Autodesk Fusion 360 part; units mm, degrees
(part 2 of 2)
  constraint tangent L245 A257
  constraint tangent A258 L248
  constraint tangent A259 L249
  constraint coincident L250.end L252
  constraint coincident L243 L250.start
  constraint horizontal L251
  constraint tangent L242 A260
  constraint tangent L251 A261
  constraint tangent L243 A261
  constraint tangent L251 A262
  constraint tangent L252 A262
  constraint tangent L247 A263
  constraint tangent L243 A263
  constraint tangent L247 A264
  constraint tangent L252 A264
  constraint coincident L252 L253.end
  constraint coincident L243 L253.start
  measures "d1" diameter of A0
  measures "d2" diameter of A1
  measures "d3" diameter of A2
  measures "d4" diameter of A3
  measures "d5" diameter of A4
  measures "d9" diameter of A111
  measures "d12" diameter of A112
  measures "d367" diameter of A246
  measures "d368" diameter of A247
  measures "d369" diameter of A248
  measures "d370" diameter of A249
extrude "Extrude1" add sketch "mriya-classic-fdm-301645" along normal blind 12.1 contours L176 L177 L198 A202 L199 A203 L200 A204 L201 A205 L202 A206 L203 A207 L204 A208 L205 A209 L206 A210 L207 L208 A212 L209 A213 L210 A214 L211 A215 L212 A216 L213 A217 L214 A218 L215 A219 L216 A220 L217 A221 L218 A222 L219 A223 L220 L221 L222 L223 L224 L225 L226 L227 L228 L229 L230 L231 L232 L233 L234 L235 L236 L237 L238 L239 L240 L241 A224 A225 A227 A228 A229 A230 A231 A232 A233 A234 A235 A236 A237 A238 A239 A240 A241 A242 A243 A244 A245 makes body 1
extrude "Extrude2" add sketch "mriya-classic-fdm-301645" along normal blind 18.6 contours L176 L177 L207 A211 L208 L235 L236 A226 bodies 1
extrude "Extrude3" add sketch "mriya-classic-fdm-301645" along normal blind 5.2 contours A114 | A115 | A116 | A117 | L198 A202 L199 A203 L200 A204 L201 A205 L202 A206 L203 A207 L204 A208 L205 A209 L206 A210 L207 L208 A212 L209 A213 L210 A214 L211 A215 L212 A216 L213 A217 L214 A218 L215 A219 L216 A220 L217 A221 L218 A222 L219 A223 L242 L244 L245 A250 A251 A252 A257 A260 | L207 A211 L208 L244 L245 A250 A251 A257 | L207 L242 A252 A260 bodies 1
extrude "Extrude13" add sketch "mriya-classic-fdm-301645" along normal blind 3.2 contours A2 | L108 L109 A118 A119 A120 L183 L184 A253 | A121 L110 A122 L111 A123 L178 L179 A254 | A124 L112 A125 L113 A126 L114 A127 L115 | A128 L116 A129 L117 A130 L118 A131 L119 | A132 L120 A133 A134 L121 L185 L186 L187 A194 A195 | A135 L122 A136 A137 L123 L180 L181 L182 A196 A197 | A138 L124 A139 L125 A140 L126 A141 L127 | A142 L128 A143 L129 A144 L130 A145 L131 | A146 L132 A147 L133 A148 L134 A149 L135 | A150 L136 A151 L137 A152 L138 A153 L139 | A154 L140 A155 L141 A156 L142 A157 L143 | A158 L144 A159 L145 A160 L146 A161 L147 | A162 L148 A163 L149 A164 L150 A165 L151 | A166 L152 A167 L153 A168 L190 L191 L192 A198 A199 | A169 L154 A170 L155 A171 L156 A172 L157 | A173 L158 A174 L159 A175 L195 L196 L197 A200 A201 | A176 L160 A177 L161 A178 L162 A179 L163 | A180 A181 L164 A182 L165 L193 L194 A256 | A183 L166 A184 L167 A185 L168 A186 L169 | A187 A188 L170 A189 L171 L188 L189 A255 | A190 L172 A191 L173 A192 L174 A193 L175 bodies 1
extrude "Extrude14" add sketch "mriya-classic-fdm-301645" along normal blind 3.2 contours A0 | A1 | A3 | A4 bodies 1
extrude "Extrude6" add sketch "mriya-classic-fdm-301645" along normal blind 1 from surface at 15.8 contours L207 A211 L208 L244 L245 A250 A251 A257 bodies 1
extrude "Extrude12" add sketch "mriya-classic-fdm-301645" along normal blind 1 from surface at 9.2 contours L207 L242 A252 A260 bodies 1
extrude "Extrude21" add sketch "mriya-classic-fdm-301645" along normal blind 2.7 contours L243 L251 L252 A261 A262 L253 | L243 L247 L250 L252 A263 A264 bodies 1
extrude "Extrude19" add sketch "mriya-classic-fdm-301645" along normal blind 1.4 contours L243 L250 L252 L253 bodies 1
sketch "power switch" plane through (-4.4, 0, 0) normal (1, 0, 0) x (0, 1, 0)
  line L0 (1.7932, 0) -> (76.6932, 0)
  line L1 (76.6932, 0) -> (76.6932, 18.6)
  line L2 (76.6932, 18.6) -> (19.2932, 18.6)
  line L3 (19.2932, 18.6) -> (19.2932, 12.1)
  line L4 (19.2932, 12.1) -> (1.7932, 12.1)
  line L5 (1.7932, 12.1) -> (1.7932, 0)
  line L6 (23.9932, 5.95) -> (23.9932, 10.8)
  line L7 (37.3932, 5.55) -> (24.3932, 5.55)
  arc A0 (37.7932, 10.8) -> (37.3932, 11.2) centre (37.3932, 10.8) ccw
  line L8 (36.0932, 9.85) -> (36.0932, 6.9)
  line L9 (25.6932, 9.85) -> (36.0932, 9.85)
  line L10 (36.0932, 6.9) -> (25.6932, 6.9)
  line L11 (25.6932, 6.9) -> (25.6932, 9.85)
  line L12 (24.3932, 11.2) -> (37.3932, 11.2)
  arc A1 (23.9932, 5.95) -> (24.3932, 5.55) centre (24.3932, 5.95) ccw
  arc A2 (37.3932, 5.55) -> (37.7932, 5.95) centre (37.3932, 5.95) ccw
  line L13 (37.7932, 10.8) -> (37.7932, 5.95)
  arc A3 (24.3932, 11.2) -> (23.9932, 10.8) centre (24.3932, 10.8) ccw
  constraint perpendicular L10 L11
  constraint vertical L11
  constraint perpendicular L9 L11
  constraint vertical L8
  constraint tangent A0 L12
  constraint tangent A0 L13
  constraint tangent A2 L13
  constraint tangent L7 A2
  constraint tangent L7 A1
  constraint tangent L6 A1
  constraint tangent L6 A3
  constraint tangent L12 A3
extrude "Extrude8" cut sketch "power switch" against normal blind 2.5 contours L8 L9 L10 L11 bodies 1
extrude "Extrude9" cut sketch "power switch" against normal blind 1 contours L6 L7 A0 L12 A1 A2 L13 A3 bodies 1
chamfer "Chamfer13" distance 1.19 angle 40 8 edges at (-4.4, 30.8932, 5.55) (-4.4, 24.1104, 5.6672) (-4.4, 23.9932, 8.375) (-4.4, 24.1104, 11.0828) (-4.4, 30.8932, 11.2) (-4.4, 37.676, 11.0828) (-4.4, 37.7932, 8.375) (-4.4, 37.676, 5.6672) measured on face at (-4.4, 63.7265, 9.8) measured on face at (-4.4, 63.7265, 9.8) measured on face at (-4.4, 63.7265, 9.8) measured on face at (-4.4, 63.7265, 9.8) measured on face at (-4.4, 63.7265, 9.8) measured on face at (-4.4, 63.7265, 9.8) measured on face at (-4.4, 63.7265, 9.8) measured on face at (-4.4, 63.7265, 9.8) on bodies 1
chamfer "Chamfer14" distance 0.5 angle 45 4 edges at (-6.9, 30.8932, 6.9) (-6.9, 25.6932, 8.375) (-6.9, 30.8932, 9.85) (-6.9, 36.0932, 8.375) on bodies 1
sketch "usb-c" plane through (0, 80.6932, 0) normal (0, 1, 0) x (-1, 0, 0)
  line L0 (8.4, 0) -> (41.0674, 0)
  line L1 (41.0674, 0) -> (41.0674, 12.1)
  line L2 (41.0674, 12.1) -> (25.8, 12.1)
  line L3 (25.8, 12.1) -> (25.8, 18.6)
  line L4 (25.8, 18.6) -> (8.4, 18.6)
  line L5 (8.4, 18.6) -> (8.4, 0)
  line L6 (19.7002, 10.3) -> (13.1003, 10.3)
  line L7 (21.8002, 14.3) -> (21.8002, 9.9)
  line L8 (21.0002, 12.6) -> (21.0002, 11.6)
  arc A0 (11.4002, 14.7) -> (11.0002, 14.3) centre (11.4002, 14.3) ccw
  arc A1 (21.4002, 9.5) -> (21.8002, 9.9) centre (21.4002, 9.9) ccw
  line L9 (11.8003, 11.6) -> (11.8003, 12.6)
  line L10 (21.4002, 9.5) -> (11.4002, 9.5)
  line L11 (11.4002, 14.7) -> (21.4002, 14.7)
  line L12 (13.1003, 13.9) -> (19.7002, 13.9)
  arc A2 (21.8002, 14.3) -> (21.4002, 14.7) centre (21.4002, 14.3) ccw
  arc A3 (11.0002, 9.9) -> (11.4002, 9.5) centre (11.4002, 9.9) ccw
  line L13 (11.0002, 9.9) -> (11.0002, 14.3)
  arc A4 (13.1003, 13.9) -> (11.8003, 12.6) centre (13.1002, 12.6) ccw
  arc A5 (11.8003, 11.6) -> (13.1003, 10.3) centre (13.1003, 11.6) ccw
  arc A6 (21.0002, 12.6) -> (19.7002, 13.9) centre (19.7002, 12.6) ccw
  arc A7 (19.7002, 10.3) -> (21.0002, 11.6) centre (19.7002, 11.6) ccw
  constraint perpendicular L7 L11
  constraint perpendicular L10 L13
  constraint horizontal L10
  constraint perpendicular L7 L10
  constraint tangent A0 L11
  constraint tangent A0 L13
  constraint tangent L11 A2
  constraint tangent L7 A2
  constraint tangent A3 L13
  constraint tangent L10 A3
  constraint tangent A1 L10
  constraint tangent L7 A1
  constraint tangent L12 A4
  constraint tangent L9 A4
  constraint tangent L9 A5
  constraint tangent L6 A5
  constraint tangent L8 A6
  constraint tangent L12 A6
  constraint tangent L6 A7
  constraint tangent L8 A7
extrude "Extrude17" cut sketch "usb-c" against normal blind 2.5 contours L6 L8 L9 L12 A4 A5 A6 A7 bodies 1
extrude "Extrude18" cut sketch "usb-c" against normal blind 1 contours L7 A0 A1 L10 L11 A2 A3 L13 bodies 1
chamfer "Chamfer23" distance 1.19 angle 40 8 edges at (-16.4003, 80.6932, 9.5) (-11.1174, 80.6932, 9.6172) (-11.0003, 80.6932, 12.1) (-11.1174, 80.6932, 14.5828) (-16.4003, 80.6932, 14.7) (-21.6831, 80.6932, 14.5828) (-21.8003, 80.6932, 12.1) (-21.6831, 80.6932, 9.6172) measured on face at (-23.6457, 80.6932, 3.1687) measured on face at (-23.6457, 80.6932, 3.1687) measured on face at (-23.6457, 80.6932, 3.1687) measured on face at (-23.6457, 80.6932, 3.1687) measured on face at (-23.6457, 80.6932, 3.1687) measured on face at (-23.6457, 80.6932, 3.1687) measured on face at (-23.6457, 80.6932, 3.1687) measured on face at (-23.6457, 80.6932, 3.1687) on bodies 1
chamfer "Chamfer21" distance 0.599 angle 45 3 edges at (-14.85, 78.1932, 15.8) (-7.3979, 77.6953, 15.8) (-6.9, 58.2432, 15.8) on bodies 1
chamfer "Chamfer22" distance 0.6 angle 45 1 edges at (-6.9, 9.5932, 9.2) on bodies 1
chamfer "Chamfer17" distance 1 angle 45 90 edges at (-17.0879, -2.2068, 12.1) (-5.5716, -1.0352, 12.1) (-4.4, 10.5432, 12.1) (-33.4337, 80.6932, 12.1) (-41.4501, 80.7693, 12.1) (-42.3387, 81.5503, 12.1) (-43.8762, 82.7648, 12.1) (-51.4458, 82.9932, 12.1) (-58.2501, 83.0693, 12.1) (-60.2387, 84.9503, 12.1) (-62.8762, 87.2648, 12.1) (-73.4, 87.4932, 12.1) (-83.9238, 87.2648, 12.1) (-86.0613, 85.4503, 12.1) (-87.5499, 84.0693, 12.1) (-94.8542, 83.9932, 12.1) (-102.9238, 83.7648, 12.1) (-107.238, 79.7735, 12.1) (-111.0657, 76.1074, 12.1) (-116.2077, 75.9932, 12.1) (-121.9238, 75.7648, 12.1) (-123.4613, 74.5503, 12.1) (-124.3499, 73.7693, 12.1) (-131.5163, 73.6932, 12.1) (-141.1284, 72.5216, 12.1) (-142.3, 42.8932, 12.1) (-141.1284, 13.2648, 12.1) (-120.4728, 12.0932, 12.1) (-100.9235, 12.4357, 12.1) (-96.4155, 16.4593, 12.1) (-92.7186, 19.941, 12.1) (-84.5898, 20.0932, 12.1) (-75.7143, 19.6842, 12.1) (-70.5474, 11.3702, 12.1) (-65.1972, 2.8703, 12.1) (-56.0828, 2.3932, 12.1) (-48.3499, 2.3171, 12.1) (-47.4613, 1.5361, 12.1) (-45.9238, 0.3216, 12.1) (-37.2542, 0.0932, 12.1) (-29.3499, 0.0171, 12.1) (-28.4613, -0.7639, 12.1) (-26.9238, -1.9784, 12.1) (-17.0879, -2.2068, 0) (-26.9238, -1.9784, 0) (-28.4613, -0.7639, 0) (-29.3499, 0.0171, 0) (-37.2542, 0.0932, 0) (-45.9238, 0.3216, 0) (-47.4613, 1.5361, 0) (-48.3499, 2.3171, 0) (-56.0828, 2.3932, 0) (-65.1972, 2.8703, 0) (-70.5474, 11.3702, 0) (-75.7143, 19.6842, 0) (-84.5898, 20.0932, 0) (-92.7186, 19.941, 0) (-96.4155, 16.4593, 0) (-100.9235, 12.4357, 0) (-120.4728, 12.0932, 0) (-141.1284, 13.2648, 0) (-142.3, 42.8932, 0) (-141.1284, 72.5216, 0) (-131.5163, 73.6932, 0) (-124.3499, 73.7693, 0) (-123.4613, 74.5503, 0) (-121.9238, 75.7648, 0) (-116.2077, 75.9932, 0) (-111.0657, 76.1074, 0) (-107.238, 79.7735, 0) (-102.9238, 83.7648, 0) (-94.8542, 83.9932, 0) (-87.5499, 84.0693, 0) (-86.0613, 85.4503, 0) (-83.9238, 87.2648, 0) (-73.4, 87.4932, 0) (-62.8762, 87.2648, 0) (-60.2387, 84.9503, 0) (-58.2501, 83.0693, 0) (-51.4458, 82.9932, 0) (-43.8762, 82.7648, 0) (-42.3387, 81.5503, 0) (-41.4501, 80.7693, 0) (-24.7337, 80.6932, 0) (-5.5716, 79.5216, 0) (-4.4, 39.2432, 0) (-5.5716, -1.0352, 0) (-4.4, 47.9932, 18.6) (-5.5716, 79.5216, 18.6) (-17.1, 80.6932, 18.6) on bodies 1
fillet "Fillet29" radius 1.2 2 edges at (-4.4, 19.2932, 14.35) (-25.8, 80.6932, 14.35) on bodies 1
chamfer "Chamfer18" distance 1 angle 45 4 edges at (-6.25, 19.2932, 18.6) (-5.4996, 19.2974, 18.6) (-25.8, 78.8432, 18.6) (-25.7958, 79.5936, 18.6) on bodies 1
chamfer "Chamfer25" distance 0.9 angle 45 6 edges at (-11.1722, 22.9091, 0) (-23.6722, 22.9091, 0) (-45.9722, 22.9591, 0) (-45.9722, 60.9591, 0) (-121.9722, 53.9591, 0) (-121.9722, 34.9591, 0) on bodies 1
sketch "silicone feets" plane through (0, 0, 0) normal (0, 0, -1) x (1, 0, 0)
  line L0 (-8.4, 1.2068) -> (-25.7757, 1.2068)
  arc A0 (-25.7757, 1.2068) -> (-27.1899, 0.621) centre (-25.7757, -0.7932) ccw
  line L1 (-27.1899, 0.621) -> (-28.3184, -0.5074)
  arc A1 (-29.7326, -1.0932) -> (-28.3184, -0.5074) centre (-29.7326, 0.9068) ccw
  line L2 (-29.7326, -1.0932) -> (-44.7757, -1.0932)
  arc A2 (-44.7757, -1.0932) -> (-46.1899, -1.679) centre (-44.7757, -3.0932) ccw
  line L3 (-46.1899, -1.679) -> (-47.3184, -2.8074)
  arc A3 (-48.7326, -3.3932) -> (-47.3184, -2.8074) centre (-48.7326, -1.3932) ccw
  line L4 (-48.7326, -3.3932) -> (-63.4331, -3.3932)
  arc A4 (-63.4331, -3.3932) -> (-65.6097, -4.6635) centre (-63.4331, -5.8932) ccw
  line L5 (-65.6097, -4.6635) -> (-73.7438, -19.0608)
  arc A5 (-77.2264, -21.0932) -> (-73.7438, -19.0608) centre (-77.2264, -17.0932) ccw
  line L6 (-77.2264, -21.0932) -> (-91.9532, -21.0932)
  arc A6 (-94.0745, -20.2145) -> (-91.9532, -21.0932) centre (-91.9532, -18.0932) ccw
  line L7 (-94.0745, -20.2145) -> (-100.1707, -14.1183)
  arc A7 (-100.1707, -14.1183) -> (-102.6456, -13.0932) centre (-102.6456, -16.5932) ccw
  line L8 (-102.6456, -13.0932) -> (-138.3, -13.0932)
  arc A8 (-138.3, -13.0932) -> (-141.3, -16.0932) centre (-138.3, -16.0932) ccw
  line L9 (-141.3, -16.0932) -> (-141.3, -69.6932)
  arc A9 (-141.3, -69.6932) -> (-138.3, -72.6932) centre (-138.3, -69.6932) ccw
  line L10 (-138.3, -72.6932) -> (-124.7326, -72.6932)
  arc A10 (-123.3184, -73.279) -> (-124.7326, -72.6932) centre (-124.7326, -74.6932) ccw
  line L11 (-123.3184, -73.279) -> (-122.1899, -74.4074)
  arc A11 (-122.1899, -74.4074) -> (-120.7757, -74.9932) centre (-120.7757, -72.9932) ccw
  line L12 (-120.7757, -74.9932) -> (-111.6397, -74.9932)
  arc A12 (-109.8719, -75.7254) -> (-111.6397, -74.9932) centre (-111.6397, -77.4932) ccw
  line L13 (-109.8719, -75.7254) -> (-103.19, -82.4074)
  arc A13 (-103.19, -82.4074) -> (-101.7757, -82.9932) centre (-101.7757, -80.9932) ccw
  line L14 (-101.7757, -82.9932) -> (-87.9326, -82.9932)
  arc A14 (-86.5184, -83.579) -> (-87.9326, -82.9932) centre (-87.9326, -84.9932) ccw
  line L15 (-86.5184, -83.579) -> (-84.19, -85.9074)
  arc A15 (-84.19, -85.9074) -> (-82.7757, -86.4932) centre (-82.7757, -84.4932) ccw
  line L16 (-82.7757, -86.4932) -> (-64.0243, -86.4932)
  arc A16 (-64.0243, -86.4932) -> (-62.6101, -85.9074) centre (-64.0243, -84.4932) ccw
  line L17 (-62.6101, -85.9074) -> (-59.2816, -82.579)
  arc A17 (-57.8674, -81.9932) -> (-59.2816, -82.579) centre (-57.8674, -83.9932) ccw
  line L18 (-57.8674, -81.9932) -> (-45.0243, -81.9932)
  arc A18 (-45.0243, -81.9932) -> (-43.6101, -81.4074) centre (-45.0243, -79.9932) ccw
  line L19 (-43.6101, -81.4074) -> (-42.4816, -80.279)
  arc A19 (-41.0674, -79.6932) -> (-42.4816, -80.279) centre (-41.0674, -81.6932) ccw
  line L20 (-41.0674, -79.6932) -> (-8.4, -79.6932)
  arc A20 (-8.4, -79.6932) -> (-5.4, -76.6932) centre (-8.4, -76.6932) ccw
  line L21 (-5.4, -76.6932) -> (-5.4, -1.7932)
  arc A21 (-5.4, -1.7932) -> (-8.4, 1.2068) centre (-8.4, -1.7932) ccw
  circle A22 centre (-11.9, -73.1932) radius 4.1
  circle A23 centre (-73.4, -79.9932) radius 4.1
  circle A24 centre (-134.8, -66.1932) radius 4.1
  circle A25 centre (-134.8, -19.5932) radius 4.1
  circle A26 centre (-61.0987, -9.8932) radius 4.1
  circle A27 centre (-11.9, -5.2932) radius 4.1
  circle A28 centre (-120.9, -53.5432) radius 2.05
  circle A29 centre (-44.9, -22.5432) radius 2.05
  circle A30 centre (-10.1, -22.4932) radius 2.05
  circle A31 centre (-22.6, -22.4932) radius 2.05
  circle A32 centre (-44.9, -60.5432) radius 2.05
  circle A33 centre (-120.9, -34.5432) radius 2.05
  dimension "d374" = 8.2
  dimension "d375" = 8.2
  dimension "d376" = 8.2
  dimension "d377" = 8.2
  dimension "d378" = 8.2
  dimension "d379" = 8.2
  dimension "d380" = 6.5
  dimension "d381" = 6.5
  dimension "d382" = 6.5
  dimension "d383" = 6.5
  dimension "d384" = 6.5
  dimension "d385" = 6.5
  dimension "d386" = 6.5
  dimension "d387" = 6.5
  dimension "d388" = 6.5
  dimension "d389" = 6.5
  dimension "d390" = 6.5
  measures "d374" diameter of A22
  measures "d375" diameter of A23
  measures "d376" diameter of A24
  measures "d377" diameter of A25
  measures "d378" diameter of A26
  measures "d379" diameter of A27
  measures "d380" distance of L20 A22.centre
  measures "d381" distance of L21 A22.centre
  measures "d382" distance of L16 A23.centre
  measures "d383" distance of L10 A24.centre
  measures "d384" distance of L9 A24.centre
  measures "d385" distance of L9 A25.centre
  measures "d386" distance of L8 A25.centre
  measures "d387" distance of L5 A26.centre
  measures "d388" distance of L4 A26.centre
  measures "d389" distance of L0 A27.centre
  measures "d390" distance of L21 A27.centre
extrude "Extrude15" cut sketch "silicone feets" against normal blind 0.8 contours A22 | A23 | A24 | A25 | A26 | A27 bodies 1
fillet "Fillet31" radius 0.8 4 edges at (-7.7, 72.0932, 2.05) (-25, 72.0932, 2.05) (-25, 24.8932, 2.05) (-7.7, 24.8932, 2.05) on bodies 1
mirror "Mirror1" about plane through (0, 0, 0) normal (1, 0, 0) of bodies 1 makes body 2
named bodies: "Left", "Right"
